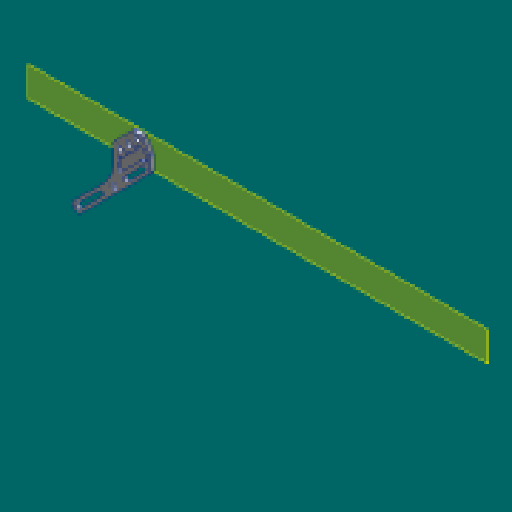
# Autodesk Inventor part: IntakeRampSidePlate
Saved by Autodesk Inventor 2023.1 (Build 271208000, 208)
## iProperties
Created: 2022-11-11
Part Number: IntakeRampSidePlate
Material: Aluminum 6061
Document SubType Name: Modeling
Designer: zac-h
Density: 2.7 g/cm^3
Appearance: Aluminum - Flat
Author: zac-h
Autodesk Inventor part; units mm, degrees
(part 1 of 2)
ref_plane "YZ Plane" through (0, 0, 0) normal (1, 0, 0) x (0, 1, 0)
ref_plane "XZ Plane" through (0, 0, 0) normal (0, 1, 0) x (-1, 0, 0)
ref_plane "XY Plane" through (0, 0, 0) normal (0, 0, 1) x (1, 0, 0)
ref_plane "Work Plane1" through (0, 0, 0) normal (0, 0, 1) x (1, 0, 0)
sketch "Sketch1" plane through (0, 0, 0) normal (0, 0, 1) x (1, 0, 0)
  line L0 (-428.9886, 23.7237) -> (-428.9886, 20.1169) projected
  arc A0 (-429.4966, 19.6089) -> (-428.9886, 20.1169) centre (-429.4966, 20.1169) ccw projected
  line L1 (-429.4966, 19.6089) -> (-433.1034, 19.6089) projected
  arc A1 (-433.6114, 20.1169) -> (-433.1034, 19.6089) centre (-433.1034, 20.1169) ccw projected
  line L2 (-433.6114, 20.1169) -> (-433.6114, 23.7237) projected
  arc A2 (-433.1034, 24.2317) -> (-433.6114, 23.7237) centre (-433.1034, 23.7237) ccw projected
  line L3 (-433.1034, 24.2317) -> (-429.4966, 24.2317) projected
  arc A3 (-428.9886, 23.7237) -> (-429.4966, 24.2317) centre (-429.4966, 23.7237) ccw projected
  line L4 (-416.2886, 23.7237) -> (-416.2886, 20.1169) projected
  arc A4 (-416.7966, 19.6089) -> (-416.2886, 20.1169) centre (-416.7966, 20.1169) ccw projected
  line L5 (-416.7966, 19.6089) -> (-420.4034, 19.6089) projected
  arc A5 (-420.9114, 20.1169) -> (-420.4034, 19.6089) centre (-420.4034, 20.1169) ccw projected
  line L6 (-420.9114, 20.1169) -> (-420.9114, 23.7237) projected
  arc A6 (-420.4034, 24.2317) -> (-420.9114, 23.7237) centre (-420.4034, 23.7237) ccw projected
  line L7 (-420.4034, 24.2317) -> (-416.7966, 24.2317) projected
  arc A7 (-416.2886, 23.7237) -> (-416.7966, 24.2317) centre (-416.7966, 23.7237) ccw projected
  line L8 (-403.5886, 23.7237) -> (-403.5886, 20.1169) projected
  arc A8 (-404.0966, 19.6089) -> (-403.5886, 20.1169) centre (-404.0966, 20.1169) ccw projected
  line L9 (-404.0966, 19.6089) -> (-407.7034, 19.6089) projected
  arc A9 (-408.2114, 20.1169) -> (-407.7034, 19.6089) centre (-407.7034, 20.1169) ccw projected
  line L10 (-408.2114, 20.1169) -> (-408.2114, 23.7237) projected
  arc A10 (-407.7034, 24.2317) -> (-408.2114, 23.7237) centre (-407.7034, 23.7237) ccw projected
  line L11 (-407.7034, 24.2317) -> (-404.0966, 24.2317) projected
  arc A11 (-403.5886, 23.7237) -> (-404.0966, 24.2317) centre (-404.0966, 23.7237) ccw projected
  line L12 (-390.8886, 23.7237) -> (-390.8886, 20.1169) projected
  arc A12 (-391.3966, 19.6089) -> (-390.8886, 20.1169) centre (-391.3966, 20.1169) ccw projected
  line L13 (-391.3966, 19.6089) -> (-395.0034, 19.6089) projected
  arc A13 (-395.5114, 20.1169) -> (-395.0034, 19.6089) centre (-395.0034, 20.1169) ccw projected
  line L14 (-395.5114, 20.1169) -> (-395.5114, 23.7237) projected
  arc A14 (-395.0034, 24.2317) -> (-395.5114, 23.7237) centre (-395.0034, 23.7237) ccw projected
  line L15 (-395.0034, 24.2317) -> (-391.3966, 24.2317) projected
  arc A15 (-390.8886, 23.7237) -> (-391.3966, 24.2317) centre (-391.3966, 23.7237) ccw projected
  line L16 (-378.1886, 23.7237) -> (-378.1886, 20.1169) projected
  arc A16 (-378.6966, 19.6089) -> (-378.1886, 20.1169) centre (-378.6966, 20.1169) ccw projected
  line L17 (-378.6966, 19.6089) -> (-382.3034, 19.6089) projected
  arc A17 (-382.8114, 20.1169) -> (-382.3034, 19.6089) centre (-382.3034, 20.1169) ccw projected
  line L18 (-382.8114, 20.1169) -> (-382.8114, 23.7237) projected
  arc A18 (-382.3034, 24.2317) -> (-382.8114, 23.7237) centre (-382.3034, 23.7237) ccw projected
  line L19 (-382.3034, 24.2317) -> (-378.6966, 24.2317) projected
  arc A19 (-378.1886, 23.7237) -> (-378.6966, 24.2317) centre (-378.6966, 23.7237) ccw projected
  line L20 (-365.4886, 23.7237) -> (-365.4886, 20.1169) projected
  arc A20 (-365.9966, 19.6089) -> (-365.4886, 20.1169) centre (-365.9966, 20.1169) ccw projected
  line L21 (-365.9966, 19.6089) -> (-369.6034, 19.6089) projected
  arc A21 (-370.1114, 20.1169) -> (-369.6034, 19.6089) centre (-369.6034, 20.1169) ccw projected
  line L22 (-370.1114, 20.1169) -> (-370.1114, 23.7237) projected
  arc A22 (-369.6034, 24.2317) -> (-370.1114, 23.7237) centre (-369.6034, 23.7237) ccw projected
  line L23 (-369.6034, 24.2317) -> (-365.9966, 24.2317) projected
  arc A23 (-365.4886, 23.7237) -> (-365.9966, 24.2317) centre (-365.9966, 23.7237) ccw projected
  line L24 (-352.7886, 23.7237) -> (-352.7886, 20.1169) projected
  arc A24 (-353.2966, 19.6089) -> (-352.7886, 20.1169) centre (-353.2966, 20.1169) ccw projected
  line L25 (-353.2966, 19.6089) -> (-356.9034, 19.6089) projected
  arc A25 (-357.4114, 20.1169) -> (-356.9034, 19.6089) centre (-356.9034, 20.1169) ccw projected
  line L26 (-357.4114, 20.1169) -> (-357.4114, 23.7237) projected
  arc A26 (-356.9034, 24.2317) -> (-357.4114, 23.7237) centre (-356.9034, 23.7237) ccw projected
  line L27 (-356.9034, 24.2317) -> (-353.2966, 24.2317) projected
  arc A27 (-352.7886, 23.7237) -> (-353.2966, 24.2317) centre (-353.2966, 23.7237) ccw projected
  line L28 (-340.0886, 23.7237) -> (-340.0886, 20.1169) projected
  arc A28 (-340.5966, 19.6089) -> (-340.0886, 20.1169) centre (-340.5966, 20.1169) ccw projected
  line L29 (-340.5966, 19.6089) -> (-344.2034, 19.6089) projected
  arc A29 (-344.7114, 20.1169) -> (-344.2034, 19.6089) centre (-344.2034, 20.1169) ccw projected
  line L30 (-344.7114, 20.1169) -> (-344.7114, 23.7237) projected
  arc A30 (-344.2034, 24.2317) -> (-344.7114, 23.7237) centre (-344.2034, 23.7237) ccw projected
  line L31 (-344.2034, 24.2317) -> (-340.5966, 24.2317) projected
  arc A31 (-340.0886, 23.7237) -> (-340.5966, 24.2317) centre (-340.5966, 23.7237) ccw projected
  line L32 (-327.3886, 23.7237) -> (-327.3886, 20.1169) projected
  arc A32 (-327.8966, 19.6089) -> (-327.3886, 20.1169) centre (-327.8966, 20.1169) ccw projected
  line L33 (-327.8966, 19.6089) -> (-331.5034, 19.6089) projected
  arc A33 (-332.0114, 20.1169) -> (-331.5034, 19.6089) centre (-331.5034, 20.1169) ccw projected
  line L34 (-332.0114, 20.1169) -> (-332.0114, 23.7237) projected
  arc A34 (-331.5034, 24.2317) -> (-332.0114, 23.7237) centre (-331.5034, 23.7237) ccw projected
  line L35 (-331.5034, 24.2317) -> (-327.8966, 24.2317) projected
  arc A35 (-327.3886, 23.7237) -> (-327.8966, 24.2317) centre (-327.8966, 23.7237) ccw projected
  line L36 (-314.6886, 23.7237) -> (-314.6886, 20.1169) projected
  arc A36 (-315.1966, 19.6089) -> (-314.6886, 20.1169) centre (-315.1966, 20.1169) ccw projected
  line L37 (-315.1966, 19.6089) -> (-318.8034, 19.6089) projected
  arc A37 (-319.3114, 20.1169) -> (-318.8034, 19.6089) centre (-318.8034, 20.1169) ccw projected
  line L38 (-319.3114, 20.1169) -> (-319.3114, 23.7237) projected
  arc A38 (-318.8034, 24.2317) -> (-319.3114, 23.7237) centre (-318.8034, 23.7237) ccw projected
  line L39 (-318.8034, 24.2317) -> (-315.1966, 24.2317) projected
  arc A39 (-314.6886, 23.7237) -> (-315.1966, 24.2317) centre (-315.1966, 23.7237) ccw projected
  line L40 (-301.9886, 23.7237) -> (-301.9886, 20.1169) projected
  arc A40 (-302.4966, 19.6089) -> (-301.9886, 20.1169) centre (-302.4966, 20.1169) ccw projected
  line L41 (-302.4966, 19.6089) -> (-306.1034, 19.6089) projected
  arc A41 (-306.6114, 20.1169) -> (-306.1034, 19.6089) centre (-306.1034, 20.1169) ccw projected
  line L42 (-306.6114, 20.1169) -> (-306.6114, 23.7237) projected
  arc A42 (-306.1034, 24.2317) -> (-306.6114, 23.7237) centre (-306.1034, 23.7237) ccw projected
  line L43 (-306.1034, 24.2317) -> (-302.4966, 24.2317) projected
  arc A43 (-301.9886, 23.7237) -> (-302.4966, 24.2317) centre (-302.4966, 23.7237) ccw projected
  line L44 (-289.2886, 23.7237) -> (-289.2886, 20.1169) projected
  arc A44 (-289.7966, 19.6089) -> (-289.2886, 20.1169) centre (-289.7966, 20.1169) ccw projected
  line L45 (-289.7966, 19.6089) -> (-293.4034, 19.6089) projected
  arc A45 (-293.9114, 20.1169) -> (-293.4034, 19.6089) centre (-293.4034, 20.1169) ccw projected
  line L46 (-293.9114, 20.1169) -> (-293.9114, 23.7237) projected
  arc A46 (-293.4034, 24.2317) -> (-293.9114, 23.7237) centre (-293.4034, 23.7237) ccw projected
  line L47 (-293.4034, 24.2317) -> (-289.7966, 24.2317) projected
  arc A47 (-289.2886, 23.7237) -> (-289.7966, 24.2317) centre (-289.7966, 23.7237) ccw projected
  line L48 (-276.5886, 23.7237) -> (-276.5886, 20.1169) projected
  arc A48 (-277.0966, 19.6089) -> (-276.5886, 20.1169) centre (-277.0966, 20.1169) ccw projected
  line L49 (-277.0966, 19.6089) -> (-280.7034, 19.6089) projected
  arc A49 (-281.2114, 20.1169) -> (-280.7034, 19.6089) centre (-280.7034, 20.1169) ccw projected
  line L50 (-281.2114, 20.1169) -> (-281.2114, 23.7237) projected
  arc A50 (-280.7034, 24.2317) -> (-281.2114, 23.7237) centre (-280.7034, 23.7237) ccw projected
  line L51 (-280.7034, 24.2317) -> (-277.0966, 24.2317) projected
  arc A51 (-276.5886, 23.7237) -> (-277.0966, 24.2317) centre (-277.0966, 23.7237) ccw projected
  line L52 (-263.8886, 23.7237) -> (-263.8886, 20.1169) projected
  arc A52 (-264.3966, 19.6089) -> (-263.8886, 20.1169) centre (-264.3966, 20.1169) ccw projected
  line L53 (-264.3966, 19.6089) -> (-268.0034, 19.6089) projected
  arc A53 (-268.5114, 20.1169) -> (-268.0034, 19.6089) centre (-268.0034, 20.1169) ccw projected
  line L54 (-268.5114, 20.1169) -> (-268.5114, 23.7237) projected
  arc A54 (-268.0034, 24.2317) -> (-268.5114, 23.7237) centre (-268.0034, 23.7237) ccw projected
  line L55 (-268.0034, 24.2317) -> (-264.3966, 24.2317) projected
  arc A55 (-263.8886, 23.7237) -> (-264.3966, 24.2317) centre (-264.3966, 23.7237) ccw projected
  line L56 (-251.1886, 23.7237) -> (-251.1886, 20.1169) projected
  arc A56 (-251.6966, 19.6089) -> (-251.1886, 20.1169) centre (-251.6966, 20.1169) ccw projected
  line L57 (-251.6966, 19.6089) -> (-255.3034, 19.6089) projected
  arc A57 (-255.8114, 20.1169) -> (-255.3034, 19.6089) centre (-255.3034, 20.1169) ccw projected
  line L58 (-255.8114, 20.1169) -> (-255.8114, 23.7237) projected
  arc A58 (-255.3034, 24.2317) -> (-255.8114, 23.7237) centre (-255.3034, 23.7237) ccw projected
  line L59 (-255.3034, 24.2317) -> (-251.6966, 24.2317) projected
  arc A59 (-251.1886, 23.7237) -> (-251.6966, 24.2317) centre (-251.6966, 23.7237) ccw projected
  line L60 (-238.4886, 23.7237) -> (-238.4886, 20.1169) projected
  arc A60 (-238.9966, 19.6089) -> (-238.4886, 20.1169) centre (-238.9966, 20.1169) ccw projected
  line L61 (-238.9966, 19.6089) -> (-242.6034, 19.6089) projected
  arc A61 (-243.1114, 20.1169) -> (-242.6034, 19.6089) centre (-242.6034, 20.1169) ccw projected
  line L62 (-243.1114, 20.1169) -> (-243.1114, 23.7237) projected
  arc A62 (-242.6034, 24.2317) -> (-243.1114, 23.7237) centre (-242.6034, 23.7237) ccw projected
  line L63 (-242.6034, 24.2317) -> (-238.9966, 24.2317) projected
  arc A63 (-238.4886, 23.7237) -> (-238.9966, 24.2317) centre (-238.9966, 23.7237) ccw projected
  line L64 (-225.7886, 23.7237) -> (-225.7886, 20.1169) projected
  arc A64 (-226.2966, 19.6089) -> (-225.7886, 20.1169) centre (-226.2966, 20.1169) ccw projected
  line L65 (-226.2966, 19.6089) -> (-229.9034, 19.6089) projected
  arc A65 (-230.4114, 20.1169) -> (-229.9034, 19.6089) centre (-229.9034, 20.1169) ccw projected
  line L66 (-230.4114, 20.1169) -> (-230.4114, 23.7237) projected
  arc A66 (-229.9034, 24.2317) -> (-230.4114, 23.7237) centre (-229.9034, 23.7237) ccw projected
  line L67 (-229.9034, 24.2317) -> (-226.2966, 24.2317) projected
  arc A67 (-225.7886, 23.7237) -> (-226.2966, 24.2317) centre (-226.2966, 23.7237) ccw projected
  line L68 (-213.0886, 23.7237) -> (-213.0886, 20.1169) projected
  arc A68 (-213.5966, 19.6089) -> (-213.0886, 20.1169) centre (-213.5966, 20.1169) ccw projected
  line L69 (-213.5966, 19.6089) -> (-217.2034, 19.6089) projected
  arc A69 (-217.7114, 20.1169) -> (-217.2034, 19.6089) centre (-217.2034, 20.1169) ccw projected
  line L70 (-217.7114, 20.1169) -> (-217.7114, 23.7237) projected
  arc A70 (-217.2034, 24.2317) -> (-217.7114, 23.7237) centre (-217.2034, 23.7237) ccw projected
  line L71 (-217.2034, 24.2317) -> (-213.5966, 24.2317) projected
  arc A71 (-213.0886, 23.7237) -> (-213.5966, 24.2317) centre (-213.5966, 23.7237) ccw projected
  line L72 (-200.3886, 23.7237) -> (-200.3886, 20.1169) projected
  arc A72 (-200.8966, 19.6089) -> (-200.3886, 20.1169) centre (-200.8966, 20.1169) ccw projected
  line L73 (-200.8966, 19.6089) -> (-204.5034, 19.6089) projected
  arc A73 (-205.0114, 20.1169) -> (-204.5034, 19.6089) centre (-204.5034, 20.1169) ccw projected
  line L74 (-205.0114, 20.1169) -> (-205.0114, 23.7237) projected
  arc A74 (-204.5034, 24.2317) -> (-205.0114, 23.7237) centre (-204.5034, 23.7237) ccw projected
  line L75 (-204.5034, 24.2317) -> (-200.8966, 24.2317) projected
  arc A75 (-200.3886, 23.7237) -> (-200.8966, 24.2317) centre (-200.8966, 23.7237) ccw projected
  line L76 (-187.6886, 23.7237) -> (-187.6886, 20.1169) projected
  arc A76 (-188.1966, 19.6089) -> (-187.6886, 20.1169) centre (-188.1966, 20.1169) ccw projected
  line L77 (-188.1966, 19.6089) -> (-191.8034, 19.6089) projected
  arc A77 (-192.3114, 20.1169) -> (-191.8034, 19.6089) centre (-191.8034, 20.1169) ccw projected
  line L78 (-192.3114, 20.1169) -> (-192.3114, 23.7237) projected
  arc A78 (-191.8034, 24.2317) -> (-192.3114, 23.7237) centre (-191.8034, 23.7237) ccw projected
  line L79 (-191.8034, 24.2317) -> (-188.1966, 24.2317) projected
  arc A79 (-187.6886, 23.7237) -> (-188.1966, 24.2317) centre (-188.1966, 23.7237) ccw projected
  line L80 (-174.9886, 23.7237) -> (-174.9886, 20.1169) projected
  arc A80 (-175.4966, 19.6089) -> (-174.9886, 20.1169) centre (-175.4966, 20.1169) ccw projected
  line L81 (-175.4966, 19.6089) -> (-179.1034, 19.6089) projected
  arc A81 (-179.6114, 20.1169) -> (-179.1034, 19.6089) centre (-179.1034, 20.1169) ccw projected
  line L82 (-179.6114, 20.1169) -> (-179.6114, 23.7237) projected
  arc A82 (-179.1034, 24.2317) -> (-179.6114, 23.7237) centre (-179.1034, 23.7237) ccw projected
  line L83 (-179.1034, 24.2317) -> (-175.4966, 24.2317) projected
  arc A83 (-174.9886, 23.7237) -> (-175.4966, 24.2317) centre (-175.4966, 23.7237) ccw projected
  line L84 (-162.2886, 23.7237) -> (-162.2886, 20.1169) projected
  arc A84 (-162.7966, 19.6089) -> (-162.2886, 20.1169) centre (-162.7966, 20.1169) ccw projected
  line L85 (-162.7966, 19.6089) -> (-166.4034, 19.6089) projected
  arc A85 (-166.9114, 20.1169) -> (-166.4034, 19.6089) centre (-166.4034, 20.1169) ccw projected
  line L86 (-166.9114, 20.1169) -> (-166.9114, 23.7237) projected
  arc A86 (-166.4034, 24.2317) -> (-166.9114, 23.7237) centre (-166.4034, 23.7237) ccw projected
  line L87 (-166.4034, 24.2317) -> (-162.7966, 24.2317) projected
  arc A87 (-162.2886, 23.7237) -> (-162.7966, 24.2317) centre (-162.7966, 23.7237) ccw projected
  line L88 (-149.5886, 23.7237) -> (-149.5886, 20.1169) projected
  arc A88 (-150.0966, 19.6089) -> (-149.5886, 20.1169) centre (-150.0966, 20.1169) ccw projected
  line L89 (-150.0966, 19.6089) -> (-153.7034, 19.6089) projected
  arc A89 (-154.2114, 20.1169) -> (-153.7034, 19.6089) centre (-153.7034, 20.1169) ccw projected
  line L90 (-154.2114, 20.1169) -> (-154.2114, 23.7237) projected
  arc A90 (-153.7034, 24.2317) -> (-154.2114, 23.7237) centre (-153.7034, 23.7237) ccw projected
  line L91 (-153.7034, 24.2317) -> (-150.0966, 24.2317) projected
  arc A91 (-149.5886, 23.7237) -> (-150.0966, 24.2317) centre (-150.0966, 23.7237) ccw projected
  line L92 (-136.8886, 23.7237) -> (-136.8886, 20.1169) projected
  arc A92 (-137.3966, 19.6089) -> (-136.8886, 20.1169) centre (-137.3966, 20.1169) ccw projected
  line L93 (-137.3966, 19.6089) -> (-141.0034, 19.6089) projected
  arc A93 (-141.5114, 20.1169) -> (-141.0034, 19.6089) centre (-141.0034, 20.1169) ccw projected
  line L94 (-141.5114, 20.1169) -> (-141.5114, 23.7237) projected
  arc A94 (-141.0034, 24.2317) -> (-141.5114, 23.7237) centre (-141.0034, 23.7237) ccw projected
  line L95 (-141.0034, 24.2317) -> (-137.3966, 24.2317) projected
  arc A95 (-136.8886, 23.7237) -> (-137.3966, 24.2317) centre (-137.3966, 23.7237) ccw projected
  line L96 (-126.5, 19.6089) -> (-126.5, 12.6321) projected
  line L97 (-126.5, 19.6089) -> (-128.3034, 19.6089) projected
  arc A96 (-128.8114, 20.1169) -> (-128.3034, 19.6089) centre (-128.3034, 20.1169) ccw projected
  line L98 (-128.8114, 20.1169) -> (-128.8114, 23.7237) projected
  arc A97 (-128.3034, 24.2317) -> (-128.8114, 23.7237) centre (-128.3034, 23.7237) ccw projected
  line L99 (-128.3034, 24.2317) -> (-126.5, 24.2317) projected
  line L100 (-126.5, 31.2085) -> (-126.5, 24.2317) projected
  line L101 (-126.5, 31.2085) -> (-127.5242, 32.2327) projected
  line L102 (-127.5242, 32.2327) -> (-188.9758, 32.2327) projected
  line L103 (-190, 31.2085) -> (-188.9758, 32.2327) projected
  line L104 (-190, 31.2085) -> (-191.0242, 32.2327) projected
  line L105 (-191.0242, 32.2327) -> (-252.4758, 32.2327) projected
  line L106 (-253.5, 31.2085) -> (-252.4758, 32.2327) projected
  line L107 (-253.5, 31.2085) -> (-254.5242, 32.2327) projected
  line L108 (-254.5242, 32.2327) -> (-315.9758, 32.2327) projected
  line L109 (-317, 31.2085) -> (-315.9758, 32.2327) projected
  line L110 (-317, 31.2085) -> (-318.0242, 32.2327) projected
  line L111 (-318.0242, 32.2327) -> (-379.4758, 32.2327) projected
  line L112 (-379.4758, 32.2327) -> (-380.5, 31.2085) projected
  line L113 (-380.5, 31.2085) -> (-381.5242, 32.2327) projected
  line L114 (-381.5242, 32.2327) -> (-444, 32.2327) projected
  line L115 (-444, 32.2327) -> (-444, 11.6079) projected
  line L116 (-444, 11.6079) -> (-381.5242, 11.6079) projected
  line L117 (-381.5242, 11.6079) -> (-380.5, 12.6321) projected
  line L118 (-380.5, 12.6321) -> (-379.4758, 11.6079) projected
  line L119 (-379.4758, 11.6079) -> (-318.0242, 11.6079) projected
  line L120 (-317, 12.6321) -> (-318.0242, 11.6079) projected
  line L121 (-317, 12.6321) -> (-315.9758, 11.6079) projected
  line L122 (-315.9758, 11.6079) -> (-254.5242, 11.6079) projected
  line L123 (-253.5, 12.6321) -> (-254.5242, 11.6079) projected
  line L124 (-253.5, 12.6321) -> (-252.4758, 11.6079) projected
  line L125 (-252.4758, 11.6079) -> (-191.0242, 11.6079) projected
  line L126 (-190, 12.6321) -> (-191.0242, 11.6079) projected
  line L127 (-190, 12.6321) -> (-188.9758, 11.6079) projected
  line L128 (-188.9758, 11.6079) -> (-127.5242, 11.6079) projected
  line L129 (-126.5, 12.6321) -> (-127.5242, 11.6079) projected
  line L130 (-435.3386, 30.0737) -> (-435.3386, 26.4669) projected
  arc A98 (-435.8466, 25.9589) -> (-435.3386, 26.4669) centre (-435.8466, 26.4669) ccw projected
  line L131 (-435.8466, 25.9589) -> (-439.4534, 25.9589) projected
  arc A99 (-439.9614, 26.4669) -> (-439.4534, 25.9589) centre (-439.4534, 26.4669) ccw projected
  line L132 (-439.9614, 26.4669) -> (-439.9614, 30.0737) projected
  arc A100 (-439.4534, 30.5817) -> (-439.9614, 30.0737) centre (-439.4534, 30.0737) ccw projected
  line L133 (-439.4534, 30.5817) -> (-435.8466, 30.5817) projected
  arc A101 (-435.3386, 30.0737) -> (-435.8466, 30.5817) centre (-435.8466, 30.0737) ccw projected
  line L134 (-435.3386, 17.3737) -> (-435.3386, 13.7669) projected
  arc A102 (-435.8466, 13.2589) -> (-435.3386, 13.7669) centre (-435.8466, 13.7669) ccw projected
  line L135 (-435.8466, 13.2589) -> (-439.4534, 13.2589) projected
  arc A103 (-439.9614, 13.7669) -> (-439.4534, 13.2589) centre (-439.4534, 13.7669) ccw projected
  line L136 (-439.9614, 13.7669) -> (-439.9614, 17.3737) projected
  arc A104 (-439.4534, 17.8817) -> (-439.9614, 17.3737) centre (-439.4534, 17.3737) ccw projected
  line L137 (-439.4534, 17.8817) -> (-435.8466, 17.8817) projected
  arc A105 (-435.3386, 17.3737) -> (-435.8466, 17.8817) centre (-435.8466, 17.3737) ccw projected
  line L138 (-427.2614, 13.7669) -> (-427.2614, 17.3737) projected
  arc A106 (-426.7534, 17.8817) -> (-427.2614, 17.3737) centre (-426.7534, 17.3737) ccw projected
  line L139 (-426.7534, 17.8817) -> (-423.1466, 17.8817) projected
  arc A107 (-422.6386, 17.3737) -> (-423.1466, 17.8817) centre (-423.1466, 17.3737) ccw projected
  line L140 (-422.6386, 17.3737) -> (-422.6386, 13.7669) projected
  arc A108 (-423.1466, 13.2589) -> (-422.6386, 13.7669) centre (-423.1466, 13.7669) ccw projected
  line L141 (-423.1466, 13.2589) -> (-426.7534, 13.2589) projected
  arc A109 (-427.2614, 13.7669) -> (-426.7534, 13.2589) centre (-426.7534, 13.7669) ccw projected
  line L142 (-414.5614, 13.7669) -> (-414.5614, 17.3737) projected
  arc A110 (-414.0534, 17.8817) -> (-414.5614, 17.3737) centre (-414.0534, 17.3737) ccw projected
  line L143 (-414.0534, 17.8817) -> (-410.4466, 17.8817) projected
  arc A111 (-409.9386, 17.3737) -> (-410.4466, 17.8817) centre (-410.4466, 17.3737) ccw projected
  line L144 (-409.9386, 17.3737) -> (-409.9386, 13.7669) projected
  arc A112 (-410.4466, 13.2589) -> (-409.9386, 13.7669) centre (-410.4466, 13.7669) ccw projected
  line L145 (-410.4466, 13.2589) -> (-414.0534, 13.2589) projected
  arc A113 (-414.5614, 13.7669) -> (-414.0534, 13.2589) centre (-414.0534, 13.7669) ccw projected
  line L146 (-401.8614, 13.7669) -> (-401.8614, 17.3737) projected
  arc A114 (-401.3534, 17.8817) -> (-401.8614, 17.3737) centre (-401.3534, 17.3737) ccw projected
  line L147 (-401.3534, 17.8817) -> (-397.7466, 17.8817) projected
  arc A115 (-397.2386, 17.3737) -> (-397.7466, 17.8817) centre (-397.7466, 17.3737) ccw projected
  line L148 (-397.2386, 17.3737) -> (-397.2386, 13.7669) projected
  arc A116 (-397.7466, 13.2589) -> (-397.2386, 13.7669) centre (-397.7466, 13.7669) ccw projected
  line L149 (-397.7466, 13.2589) -> (-401.3534, 13.2589) projected
  arc A117 (-401.8614, 13.7669) -> (-401.3534, 13.2589) centre (-401.3534, 13.7669) ccw projected
  line L150 (-389.1614, 13.7669) -> (-389.1614, 17.3737) projected
  arc A118 (-388.6534, 17.8817) -> (-389.1614, 17.3737) centre (-388.6534, 17.3737) ccw projected
  line L151 (-388.6534, 17.8817) -> (-385.0466, 17.8817) projected
  arc A119 (-384.5386, 17.3737) -> (-385.0466, 17.8817) centre (-385.0466, 17.3737) ccw projected
  line L152 (-384.5386, 17.3737) -> (-384.5386, 13.7669) projected
  arc A120 (-385.0466, 13.2589) -> (-384.5386, 13.7669) centre (-385.0466, 13.7669) ccw projected
  line L153 (-385.0466, 13.2589) -> (-388.6534, 13.2589) projected
  arc A121 (-389.1614, 13.7669) -> (-388.6534, 13.2589) centre (-388.6534, 13.7669) ccw projected
  line L154 (-376.4614, 13.7669) -> (-376.4614, 17.3737) projected
  arc A122 (-375.9534, 17.8817) -> (-376.4614, 17.3737) centre (-375.9534, 17.3737) ccw projected
  line L155 (-375.9534, 17.8817) -> (-372.3466, 17.8817) projected
  arc A123 (-371.8386, 17.3737) -> (-372.3466, 17.8817) centre (-372.3466, 17.3737) ccw projected
  line L156 (-371.8386, 17.3737) -> (-371.8386, 13.7669) projected
  arc A124 (-372.3466, 13.2589) -> (-371.8386, 13.7669) centre (-372.3466, 13.7669) ccw projected
  line L157 (-372.3466, 13.2589) -> (-375.9534, 13.2589) projected
  arc A125 (-376.4614, 13.7669) -> (-375.9534, 13.2589) centre (-375.9534, 13.7669) ccw projected
  line L158 (-363.7614, 13.7669) -> (-363.7614, 17.3737) projected
  arc A126 (-363.2534, 17.8817) -> (-363.7614, 17.3737) centre (-363.2534, 17.3737) ccw projected
  line L159 (-363.2534, 17.8817) -> (-359.6466, 17.8817) projected
  arc A127 (-359.1386, 17.3737) -> (-359.6466, 17.8817) centre (-359.6466, 17.3737) ccw projected
  line L160 (-359.1386, 17.3737) -> (-359.1386, 13.7669) projected
  arc A128 (-359.6466, 13.2589) -> (-359.1386, 13.7669) centre (-359.6466, 13.7669) ccw projected
  line L161 (-359.6466, 13.2589) -> (-363.2534, 13.2589) projected
  arc A129 (-363.7614, 13.7669) -> (-363.2534, 13.2589) centre (-363.2534, 13.7669) ccw projected
  line L162 (-351.0614, 13.7669) -> (-351.0614, 17.3737) projected
  arc A130 (-350.5534, 17.8817) -> (-351.0614, 17.3737) centre (-350.5534, 17.3737) ccw projected
  line L163 (-350.5534, 17.8817) -> (-346.9466, 17.8817) projected
  arc A131 (-346.4386, 17.3737) -> (-346.9466, 17.8817) centre (-346.9466, 17.3737) ccw projected
  line L164 (-346.4386, 17.3737) -> (-346.4386, 13.7669) projected
  arc A132 (-346.9466, 13.2589) -> (-346.4386, 13.7669) centre (-346.9466, 13.7669) ccw projected
  line L165 (-346.9466, 13.2589) -> (-350.5534, 13.2589) projected
  arc A133 (-351.0614, 13.7669) -> (-350.5534, 13.2589) centre (-350.5534, 13.7669) ccw projected
  line L166 (-338.3614, 13.7669) -> (-338.3614, 17.3737) projected
  arc A134 (-337.8534, 17.8817) -> (-338.3614, 17.3737) centre (-337.8534, 17.3737) ccw projected
  line L167 (-337.8534, 17.8817) -> (-334.2466, 17.8817) projected
  arc A135 (-333.7386, 17.3737) -> (-334.2466, 17.8817) centre (-334.2466, 17.3737) ccw projected
  line L168 (-333.7386, 17.3737) -> (-333.7386, 13.7669) projected
  arc A136 (-334.2466, 13.2589) -> (-333.7386, 13.7669) centre (-334.2466, 13.7669) ccw projected
  line L169 (-334.2466, 13.2589) -> (-337.8534, 13.2589) projected
  arc A137 (-338.3614, 13.7669) -> (-337.8534, 13.2589) centre (-337.8534, 13.7669) ccw projected
  line L170 (-325.6614, 13.7669) -> (-325.6614, 17.3737) projected
  arc A138 (-325.1534, 17.8817) -> (-325.6614, 17.3737) centre (-325.1534, 17.3737) ccw projected
  line L171 (-325.1534, 17.8817) -> (-321.5466, 17.8817) projected
  arc A139 (-321.0386, 17.3737) -> (-321.5466, 17.8817) centre (-321.5466, 17.3737) ccw projected
  line L172 (-321.0386, 17.3737) -> (-321.0386, 13.7669) projected
  arc A140 (-321.5466, 13.2589) -> (-321.0386, 13.7669) centre (-321.5466, 13.7669) ccw projected
  line L173 (-321.5466, 13.2589) -> (-325.1534, 13.2589) projected
  arc A141 (-325.6614, 13.7669) -> (-325.1534, 13.2589) centre (-325.1534, 13.7669) ccw projected
  line L174 (-312.9614, 13.7669) -> (-312.9614, 17.3737) projected
  arc A142 (-312.4534, 17.8817) -> (-312.9614, 17.3737) centre (-312.4534, 17.3737) ccw projected
  line L175 (-312.4534, 17.8817) -> (-308.8466, 17.8817) projected
  arc A143 (-308.3386, 17.3737) -> (-308.8466, 17.8817) centre (-308.8466, 17.3737) ccw projected
  line L176 (-308.3386, 17.3737) -> (-308.3386, 13.7669) projected
  arc A144 (-308.8466, 13.2589) -> (-308.3386, 13.7669) centre (-308.8466, 13.7669) ccw projected
  line L177 (-308.8466, 13.2589) -> (-312.4534, 13.2589) projected
  arc A145 (-312.9614, 13.7669) -> (-312.4534, 13.2589) centre (-312.4534, 13.7669) ccw projected
  line L178 (-300.2614, 13.7669) -> (-300.2614, 17.3737) projected
  arc A146 (-299.7534, 17.8817) -> (-300.2614, 17.3737) centre (-299.7534, 17.3737) ccw projected
  line L179 (-299.7534, 17.8817) -> (-296.1466, 17.8817) projected
  arc A147 (-295.6386, 17.3737) -> (-296.1466, 17.8817) centre (-296.1466, 17.3737) ccw projected
  line L180 (-295.6386, 17.3737) -> (-295.6386, 13.7669) projected
  arc A148 (-296.1466, 13.2589) -> (-295.6386, 13.7669) centre (-296.1466, 13.7669) ccw projected
  line L181 (-296.1466, 13.2589) -> (-299.7534, 13.2589) projected
  arc A149 (-300.2614, 13.7669) -> (-299.7534, 13.2589) centre (-299.7534, 13.7669) ccw projected
  line L182 (-287.5614, 13.7669) -> (-287.5614, 17.3737) projected
  arc A150 (-287.0534, 17.8817) -> (-287.5614, 17.3737) centre (-287.0534, 17.3737) ccw projected
  line L183 (-287.0534, 17.8817) -> (-283.4466, 17.8817) projected
  arc A151 (-282.9386, 17.3737) -> (-283.4466, 17.8817) centre (-283.4466, 17.3737) ccw projected
  line L184 (-282.9386, 17.3737) -> (-282.9386, 13.7669) projected
  arc A152 (-283.4466, 13.2589) -> (-282.9386, 13.7669) centre (-283.4466, 13.7669) ccw projected
  line L185 (-283.4466, 13.2589) -> (-287.0534, 13.2589) projected
  arc A153 (-287.5614, 13.7669) -> (-287.0534, 13.2589) centre (-287.0534, 13.7669) ccw projected
  line L186 (-274.8614, 13.7669) -> (-274.8614, 17.3737) projected
  arc A154 (-274.3534, 17.8817) -> (-274.8614, 17.3737) centre (-274.3534, 17.3737) ccw projected
  line L187 (-274.3534, 17.8817) -> (-270.7466, 17.8817) projected
  arc A155 (-270.2386, 17.3737) -> (-270.7466, 17.8817) centre (-270.7466, 17.3737) ccw projected
  line L188 (-270.2386, 17.3737) -> (-270.2386, 13.7669) projected
  arc A156 (-270.7466, 13.2589) -> (-270.2386, 13.7669) centre (-270.7466, 13.7669) ccw projected
  line L189 (-270.7466, 13.2589) -> (-274.3534, 13.2589) projected
  arc A157 (-274.8614, 13.7669) -> (-274.3534, 13.2589) centre (-274.3534, 13.7669) ccw projected
  line L190 (-262.1614, 13.7669) -> (-262.1614, 17.3737) projected
  arc A158 (-261.6534, 17.8817) -> (-262.1614, 17.3737) centre (-261.6534, 17.3737) ccw projected
  line L191 (-261.6534, 17.8817) -> (-258.0466, 17.8817) projected
  arc A159 (-257.5386, 17.3737) -> (-258.0466, 17.8817) centre (-258.0466, 17.3737) ccw projected
  line L192 (-257.5386, 17.3737) -> (-257.5386, 13.7669) projected
  arc A160 (-258.0466, 13.2589) -> (-257.5386, 13.7669) centre (-258.0466, 13.7669) ccw projected
  line L193 (-258.0466, 13.2589) -> (-261.6534, 13.2589) projected
  arc A161 (-262.1614, 13.7669) -> (-261.6534, 13.2589) centre (-261.6534, 13.7669) ccw projected
  line L194 (-249.4614, 13.7669) -> (-249.4614, 17.3737) projected
  arc A162 (-248.9534, 17.8817) -> (-249.4614, 17.3737) centre (-248.9534, 17.3737) ccw projected
  line L195 (-248.9534, 17.8817) -> (-245.3466, 17.8817) projected
  arc A163 (-244.8386, 17.3737) -> (-245.3466, 17.8817) centre (-245.3466, 17.3737) ccw projected
  line L196 (-244.8386, 17.3737) -> (-244.8386, 13.7669) projected
  arc A164 (-245.3466, 13.2589) -> (-244.8386, 13.7669) centre (-245.3466, 13.7669) ccw projected
  line L197 (-245.3466, 13.2589) -> (-248.9534, 13.2589) projected
  arc A165 (-249.4614, 13.7669) -> (-248.9534, 13.2589) centre (-248.9534, 13.7669) ccw projected
  line L198 (-236.7614, 13.7669) -> (-236.7614, 17.3737) projected
  arc A166 (-236.2534, 17.8817) -> (-236.7614, 17.3737) centre (-236.2534, 17.3737) ccw projected
  line L199 (-236.2534, 17.8817) -> (-232.6466, 17.8817) projected
  arc A167 (-232.1386, 17.3737) -> (-232.6466, 17.8817) centre (-232.6466, 17.3737) ccw projected
  line L200 (-232.1386, 17.3737) -> (-232.1386, 13.7669) projected
  arc A168 (-232.6466, 13.2589) -> (-232.1386, 13.7669) centre (-232.6466, 13.7669) ccw projected
  line L201 (-232.6466, 13.2589) -> (-236.2534, 13.2589) projected
  arc A169 (-236.7614, 13.7669) -> (-236.2534, 13.2589) centre (-236.2534, 13.7669) ccw projected
  line L202 (-224.0614, 13.7669) -> (-224.0614, 17.3737) projected
  arc A170 (-223.5534, 17.8817) -> (-224.0614, 17.3737) centre (-223.5534, 17.3737) ccw projected
  line L203 (-223.5534, 17.8817) -> (-219.9466, 17.8817) projected
  arc A171 (-219.4386, 17.3737) -> (-219.9466, 17.8817) centre (-219.9466, 17.3737) ccw projected
  line L204 (-219.4386, 17.3737) -> (-219.4386, 13.7669) projected
  arc A172 (-219.9466, 13.2589) -> (-219.4386, 13.7669) centre (-219.9466, 13.7669) ccw projected
  line L205 (-219.9466, 13.2589) -> (-223.5534, 13.2589) projected
  arc A173 (-224.0614, 13.7669) -> (-223.5534, 13.2589) centre (-223.5534, 13.7669) ccw projected
  line L206 (-211.3614, 13.7669) -> (-211.3614, 17.3737) projected
  arc A174 (-210.8534, 17.8817) -> (-211.3614, 17.3737) centre (-210.8534, 17.3737) ccw projected
  line L207 (-210.8534, 17.8817) -> (-207.2466, 17.8817) projected
  arc A175 (-206.7386, 17.3737) -> (-207.2466, 17.8817) centre (-207.2466, 17.3737) ccw projected
  line L208 (-206.7386, 17.3737) -> (-206.7386, 13.7669) projected
  arc A176 (-207.2466, 13.2589) -> (-206.7386, 13.7669) centre (-207.2466, 13.7669) ccw projected
  line L209 (-207.2466, 13.2589) -> (-210.8534, 13.2589) projected
  arc A177 (-211.3614, 13.7669) -> (-210.8534, 13.2589) centre (-210.8534, 13.7669) ccw projected
  line L210 (-198.6614, 13.7669) -> (-198.6614, 17.3737) projected
  arc A178 (-198.1534, 17.8817) -> (-198.6614, 17.3737) centre (-198.1534, 17.3737) ccw projected
  line L211 (-198.1534, 17.8817) -> (-194.5466, 17.8817) projected
  arc A179 (-194.0386, 17.3737) -> (-194.5466, 17.8817) centre (-194.5466, 17.3737) ccw projected
  line L212 (-194.0386, 17.3737) -> (-194.0386, 13.7669) projected
  arc A180 (-194.5466, 13.2589) -> (-194.0386, 13.7669) centre (-194.5466, 13.7669) ccw projected
  line L213 (-194.5466, 13.2589) -> (-198.1534, 13.2589) projected
  arc A181 (-198.6614, 13.7669) -> (-198.1534, 13.2589) centre (-198.1534, 13.7669) ccw projected
  line L214 (-185.9614, 13.7669) -> (-185.9614, 17.3737) projected
  arc A182 (-185.4534, 17.8817) -> (-185.9614, 17.3737) centre (-185.4534, 17.3737) ccw projected
  line L215 (-185.4534, 17.8817) -> (-181.8466, 17.8817) projected
  arc A183 (-181.3386, 17.3737) -> (-181.8466, 17.8817) centre (-181.8466, 17.3737) ccw projected
  line L216 (-181.3386, 17.3737) -> (-181.3386, 13.7669) projected
  arc A184 (-181.8466, 13.2589) -> (-181.3386, 13.7669) centre (-181.8466, 13.7669) ccw projected
  line L217 (-181.8466, 13.2589) -> (-185.4534, 13.2589) projected
  arc A185 (-185.9614, 13.7669) -> (-185.4534, 13.2589) centre (-185.4534, 13.7669) ccw projected
  line L218 (-173.2614, 13.7669) -> (-173.2614, 17.3737) projected
  arc A186 (-172.7534, 17.8817) -> (-173.2614, 17.3737) centre (-172.7534, 17.3737) ccw projected
  line L219 (-172.7534, 17.8817) -> (-169.1466, 17.8817) projected
  arc A187 (-168.6386, 17.3737) -> (-169.1466, 17.8817) centre (-169.1466, 17.3737) ccw projected
  line L220 (-168.6386, 17.3737) -> (-168.6386, 13.7669) projected
  arc A188 (-169.1466, 13.2589) -> (-168.6386, 13.7669) centre (-169.1466, 13.7669) ccw projected
  line L221 (-169.1466, 13.2589) -> (-172.7534, 13.2589) projected
  arc A189 (-173.2614, 13.7669) -> (-172.7534, 13.2589) centre (-172.7534, 13.7669) ccw projected
  line L222 (-160.5614, 13.7669) -> (-160.5614, 17.3737) projected
  arc A190 (-160.0534, 17.8817) -> (-160.5614, 17.3737) centre (-160.0534, 17.3737) ccw projected
  line L223 (-160.0534, 17.8817) -> (-156.4466, 17.8817) projected
  arc A191 (-155.9386, 17.3737) -> (-156.4466, 17.8817) centre (-156.4466, 17.3737) ccw projected
  line L224 (-155.9386, 17.3737) -> (-155.9386, 13.7669) projected
  arc A192 (-156.4466, 13.2589) -> (-155.9386, 13.7669) centre (-156.4466, 13.7669) ccw projected
  line L225 (-156.4466, 13.2589) -> (-160.0534, 13.2589) projected
  arc A193 (-160.5614, 13.7669) -> (-160.0534, 13.2589) centre (-160.0534, 13.7669) ccw projected
  line L226 (-147.8614, 13.7669) -> (-147.8614, 17.3737) projected
  arc A194 (-147.3534, 17.8817) -> (-147.8614, 17.3737) centre (-147.3534, 17.3737) ccw projected
  line L227 (-147.3534, 17.8817) -> (-143.7466, 17.8817) projected
  arc A195 (-143.2386, 17.3737) -> (-143.7466, 17.8817) centre (-143.7466, 17.3737) ccw projected
  line L228 (-143.2386, 17.3737) -> (-143.2386, 13.7669) projected
  arc A196 (-143.7466, 13.2589) -> (-143.2386, 13.7669) centre (-143.7466, 13.7669) ccw projected
  line L229 (-143.7466, 13.2589) -> (-147.3534, 13.2589) projected
  arc A197 (-147.8614, 13.7669) -> (-147.3534, 13.2589) centre (-147.3534, 13.7669) ccw projected
  line L230 (-135.1614, 13.7669) -> (-135.1614, 17.3737) projected
  arc A198 (-134.6534, 17.8817) -> (-135.1614, 17.3737) centre (-134.6534, 17.3737) ccw projected
  line L231 (-134.6534, 17.8817) -> (-131.0466, 17.8817) projected
  arc A199 (-130.5386, 17.3737) -> (-131.0466, 17.8817) centre (-131.0466, 17.3737) ccw projected
  line L232 (-130.5386, 17.3737) -> (-130.5386, 13.7669) projected
  arc A200 (-131.0466, 13.2589) -> (-130.5386, 13.7669) centre (-131.0466, 13.7669) ccw projected
  line L233 (-131.0466, 13.2589) -> (-134.6534, 13.2589) projected
  arc A201 (-135.1614, 13.7669) -> (-134.6534, 13.2589) centre (-134.6534, 13.7669) ccw projected
  line L234 (-427.2614, 26.4669) -> (-427.2614, 30.0737) projected
  arc A202 (-426.7534, 30.5817) -> (-427.2614, 30.0737) centre (-426.7534, 30.0737) ccw projected
  line L235 (-426.7534, 30.5817) -> (-423.1466, 30.5817) projected
  arc A203 (-422.6386, 30.0737) -> (-423.1466, 30.5817) centre (-423.1466, 30.0737) ccw projected
  line L236 (-422.6386, 30.0737) -> (-422.6386, 26.4669) projected
  arc A204 (-423.1466, 25.9589) -> (-422.6386, 26.4669) centre (-423.1466, 26.4669) ccw projected
  line L237 (-423.1466, 25.9589) -> (-426.7534, 25.9589) projected
  arc A205 (-427.2614, 26.4669) -> (-426.7534, 25.9589) centre (-426.7534, 26.4669) ccw projected
  line L238 (-414.5614, 26.4669) -> (-414.5614, 30.0737) projected
  arc A206 (-414.0534, 30.5817) -> (-414.5614, 30.0737) centre (-414.0534, 30.0737) ccw projected
  line L239 (-414.0534, 30.5817) -> (-410.4466, 30.5817) projected
  arc A207 (-409.9386, 30.0737) -> (-410.4466, 30.5817) centre (-410.4466, 30.0737) ccw projected
  line L240 (-409.9386, 30.0737) -> (-409.9386, 26.4669) projected
  arc A208 (-410.4466, 25.9589) -> (-409.9386, 26.4669) centre (-410.4466, 26.4669) ccw projected
  line L241 (-410.4466, 25.9589) -> (-414.0534, 25.9589) projected
  arc A209 (-414.5614, 26.4669) -> (-414.0534, 25.9589) centre (-414.0534, 26.4669) ccw projected
  line L242 (-401.8614, 26.4669) -> (-401.8614, 30.0737) projected
  arc A210 (-401.3534, 30.5817) -> (-401.8614, 30.0737) centre (-401.3534, 30.0737) ccw projected
  line L243 (-401.3534, 30.5817) -> (-397.7466, 30.5817) projected
  arc A211 (-397.2386, 30.0737) -> (-397.7466, 30.5817) centre (-397.7466, 30.0737) ccw projected
  line L244 (-397.2386, 30.0737) -> (-397.2386, 26.4669) projected
  arc A212 (-397.7466, 25.9589) -> (-397.2386, 26.4669) centre (-397.7466, 26.4669) ccw projected
  line L245 (-397.7466, 25.9589) -> (-401.3534, 25.9589) projected
  arc A213 (-401.8614, 26.4669) -> (-401.3534, 25.9589) centre (-401.3534, 26.4669) ccw projected
  line L246 (-389.1614, 26.4669) -> (-389.1614, 30.0737) projected
  arc A214 (-388.6534, 30.5817) -> (-389.1614, 30.0737) centre (-388.6534, 30.0737) ccw projected
  line L247 (-388.6534, 30.5817) -> (-385.0466, 30.5817) projected
  arc A215 (-384.5386, 30.0737) -> (-385.0466, 30.5817) centre (-385.0466, 30.0737) ccw projected
  line L248 (-384.5386, 30.0737) -> (-384.5386, 26.4669) projected
  arc A216 (-385.0466, 25.9589) -> (-384.5386, 26.4669) centre (-385.0466, 26.4669) ccw projected
  line L249 (-385.0466, 25.9589) -> (-388.6534, 25.9589) projected
  arc A217 (-389.1614, 26.4669) -> (-388.6534, 25.9589) centre (-388.6534, 26.4669) ccw projected
  line L250 (-376.4614, 26.4669) -> (-376.4614, 30.0737) projected
  arc A218 (-375.9534, 30.5817) -> (-376.4614, 30.0737) centre (-375.9534, 30.0737) ccw projected
  line L251 (-375.9534, 30.5817) -> (-372.3466, 30.5817) projected
  arc A219 (-371.8386, 30.0737) -> (-372.3466, 30.5817) centre (-372.3466, 30.0737) ccw projected
  line L252 (-371.8386, 30.0737) -> (-371.8386, 26.4669) projected
  arc A220 (-372.3466, 25.9589) -> (-371.8386, 26.4669) centre (-372.3466, 26.4669) ccw projected
  line L253 (-372.3466, 25.9589) -> (-375.9534, 25.9589) projected
  arc A221 (-376.4614, 26.4669) -> (-375.9534, 25.9589) centre (-375.9534, 26.4669) ccw projected
  line L254 (-363.7614, 26.4669) -> (-363.7614, 30.0737) projected
  arc A222 (-363.2534, 30.5817) -> (-363.7614, 30.0737) centre (-363.2534, 30.0737) ccw projected
  line L255 (-363.2534, 30.5817) -> (-359.6466, 30.5817) projected
  arc A223 (-359.1386, 30.0737) -> (-359.6466, 30.5817) centre (-359.6466, 30.0737) ccw projected
  line L256 (-359.1386, 30.0737) -> (-359.1386, 26.4669) projected
  arc A224 (-359.6466, 25.9589) -> (-359.1386, 26.4669) centre (-359.6466, 26.4669) ccw projected
  line L257 (-359.6466, 25.9589) -> (-363.2534, 25.9589) projected
  arc A225 (-363.7614, 26.4669) -> (-363.2534, 25.9589) centre (-363.2534, 26.4669) ccw projected
  line L258 (-351.0614, 26.4669) -> (-351.0614, 30.0737) projected
  arc A226 (-350.5534, 30.5817) -> (-351.0614, 30.0737) centre (-350.5534, 30.0737) ccw projected
  line L259 (-350.5534, 30.5817) -> (-346.9466, 30.5817) projected
  arc A227 (-346.4386, 30.0737) -> (-346.9466, 30.5817) centre (-346.9466, 30.0737) ccw projected
  line L260 (-346.4386, 30.0737) -> (-346.4386, 26.4669) projected
  arc A228 (-346.9466, 25.9589) -> (-346.4386, 26.4669) centre (-346.9466, 26.4669) ccw projected
  line L261 (-346.9466, 25.9589) -> (-350.5534, 25.9589) projected
  arc A229 (-351.0614, 26.4669) -> (-350.5534, 25.9589) centre (-350.5534, 26.4669) ccw projected
  line L262 (-338.3614, 26.4669) -> (-338.3614, 30.0737) projected
  arc A230 (-337.8534, 30.5817) -> (-338.3614, 30.0737) centre (-337.8534, 30.0737) ccw projected
  line L263 (-337.8534, 30.5817) -> (-334.2466, 30.5817) projected
  arc A231 (-333.7386, 30.0737) -> (-334.2466, 30.5817) centre (-334.2466, 30.0737) ccw projected
  line L264 (-333.7386, 30.0737) -> (-333.7386, 26.4669) projected
  arc A232 (-334.2466, 25.9589) -> (-333.7386, 26.4669) centre (-334.2466, 26.4669) ccw projected
  line L265 (-334.2466, 25.9589) -> (-337.8534, 25.9589) projected
  arc A233 (-338.3614, 26.4669) -> (-337.8534, 25.9589) centre (-337.8534, 26.4669) ccw projected
  line L266 (-325.6614, 26.4669) -> (-325.6614, 30.0737) projected
  arc A234 (-325.1534, 30.5817) -> (-325.6614, 30.0737) centre (-325.1534, 30.0737) ccw projected
  line L267 (-325.1534, 30.5817) -> (-321.5466, 30.5817) projected
  arc A235 (-321.0386, 30.0737) -> (-321.5466, 30.5817) centre (-321.5466, 30.0737) ccw projected
  line L268 (-321.0386, 30.0737) -> (-321.0386, 26.4669) projected
  arc A236 (-321.5466, 25.9589) -> (-321.0386, 26.4669) centre (-321.5466, 26.4669) ccw projected
  line L269 (-321.5466, 25.9589) -> (-325.1534, 25.9589) projected
  arc A237 (-325.6614, 26.4669) -> (-325.1534, 25.9589) centre (-325.1534, 26.4669) ccw projected
  line L270 (-312.9614, 26.4669) -> (-312.9614, 30.0737) projected
  arc A238 (-312.4534, 30.5817) -> (-312.9614, 30.0737) centre (-312.4534, 30.0737) ccw projected
  line L271 (-312.4534, 30.5817) -> (-308.8466, 30.5817) projected
  arc A239 (-308.3386, 30.0737) -> (-308.8466, 30.5817) centre (-308.8466, 30.0737) ccw projected
  line L272 (-308.3386, 30.0737) -> (-308.3386, 26.4669) projected
  arc A240 (-308.8466, 25.9589) -> (-308.3386, 26.4669) centre (-308.8466, 26.4669) ccw projected
  line L273 (-308.8466, 25.9589) -> (-312.4534, 25.9589) projected
  arc A241 (-312.9614, 26.4669) -> (-312.4534, 25.9589) centre (-312.4534, 26.4669) ccw projected
  line L274 (-300.2614, 26.4669) -> (-300.2614, 30.0737) projected
  arc A242 (-299.7534, 30.5817) -> (-300.2614, 30.0737) centre (-299.7534, 30.0737) ccw projected
  line L275 (-299.7534, 30.5817) -> (-296.1466, 30.5817) projected
  arc A243 (-295.6386, 30.0737) -> (-296.1466, 30.5817) centre (-296.1466, 30.0737) ccw projected
  line L276 (-295.6386, 30.0737) -> (-295.6386, 26.4669) projected
  arc A244 (-296.1466, 25.9589) -> (-295.6386, 26.4669) centre (-296.1466, 26.4669) ccw projected
  line L277 (-296.1466, 25.9589) -> (-299.7534, 25.9589) projected
  arc A245 (-300.2614, 26.4669) -> (-299.7534, 25.9589) centre (-299.7534, 26.4669) ccw projected
  line L278 (-287.5614, 26.4669) -> (-287.5614, 30.0737) projected
  arc A246 (-287.0534, 30.5817) -> (-287.5614, 30.0737) centre (-287.0534, 30.0737) ccw projected
  line L279 (-287.0534, 30.5817) -> (-283.4466, 30.5817) projected
  arc A247 (-282.9386, 30.0737) -> (-283.4466, 30.5817) centre (-283.4466, 30.0737) ccw projected
  line L280 (-282.9386, 30.0737) -> (-282.9386, 26.4669) projected
  arc A248 (-283.4466, 25.9589) -> (-282.9386, 26.4669) centre (-283.4466, 26.4669) ccw projected
  line L281 (-283.4466, 25.9589) -> (-287.0534, 25.9589) projected
  arc A249 (-287.5614, 26.4669) -> (-287.0534, 25.9589) centre (-287.0534, 26.4669) ccw projected
  line L282 (-274.8614, 26.4669) -> (-274.8614, 30.0737) projected
  arc A250 (-274.3534, 30.5817) -> (-274.8614, 30.0737) centre (-274.3534, 30.0737) ccw projected
  line L283 (-274.3534, 30.5817) -> (-270.7466, 30.5817) projected
  arc A251 (-270.2386, 30.0737) -> (-270.7466, 30.5817) centre (-270.7466, 30.0737) ccw projected
  line L284 (-270.2386, 30.0737) -> (-270.2386, 26.4669) projected
  arc A252 (-270.7466, 25.9589) -> (-270.2386, 26.4669) centre (-270.7466, 26.4669) ccw projected
  line L285 (-270.7466, 25.9589) -> (-274.3534, 25.9589) projected
  arc A253 (-274.8614, 26.4669) -> (-274.3534, 25.9589) centre (-274.3534, 26.4669) ccw projected
  line L286 (-262.1614, 26.4669) -> (-262.1614, 30.0737) projected
  arc A254 (-261.6534, 30.5817) -> (-262.1614, 30.0737) centre (-261.6534, 30.0737) ccw projected
  line L287 (-261.6534, 30.5817) -> (-258.0466, 30.5817) projected
  arc A255 (-257.5386, 30.0737) -> (-258.0466, 30.5817) centre (-258.0466, 30.0737) ccw projected
  line L288 (-257.5386, 30.0737) -> (-257.5386, 26.4669) projected
  arc A256 (-258.0466, 25.9589) -> (-257.5386, 26.4669) centre (-258.0466, 26.4669) ccw projected
  line L289 (-258.0466, 25.9589) -> (-261.6534, 25.9589) projected
  arc A257 (-262.1614, 26.4669) -> (-261.6534, 25.9589) centre (-261.6534, 26.4669) ccw projected
  line L290 (-249.4614, 26.4669) -> (-249.4614, 30.0737) projected
  arc A258 (-248.9534, 30.5817) -> (-249.4614, 30.0737) centre (-248.9534, 30.0737) ccw projected
  line L291 (-248.9534, 30.5817) -> (-245.3466, 30.5817) projected
  arc A259 (-244.8386, 30.0737) -> (-245.3466, 30.5817) centre (-245.3466, 30.0737) ccw projected
  line L292 (-244.8386, 30.0737) -> (-244.8386, 26.4669) projected
  arc A260 (-245.3466, 25.9589) -> (-244.8386, 26.4669) centre (-245.3466, 26.4669) ccw projected
  line L293 (-245.3466, 25.9589) -> (-248.9534, 25.9589) projected
  arc A261 (-249.4614, 26.4669) -> (-248.9534, 25.9589) centre (-248.9534, 26.4669) ccw projected
  line L294 (-236.7614, 26.4669) -> (-236.7614, 30.0737) projected
  arc A262 (-236.2534, 30.5817) -> (-236.7614, 30.0737) centre (-236.2534, 30.0737) ccw projected
  line L295 (-236.2534, 30.5817) -> (-232.6466, 30.5817) projected
  arc A263 (-232.1386, 30.0737) -> (-232.6466, 30.5817) centre (-232.6466, 30.0737) ccw projected
  line L296 (-232.1386, 30.0737) -> (-232.1386, 26.4669) projected
  arc A264 (-232.6466, 25.9589) -> (-232.1386, 26.4669) centre (-232.6466, 26.4669) ccw projected
  line L297 (-232.6466, 25.9589) -> (-236.2534, 25.9589) projected
  arc A265 (-236.7614, 26.4669) -> (-236.2534, 25.9589) centre (-236.2534, 26.4669) ccw projected
  line L298 (-224.0614, 26.4669) -> (-224.0614, 30.0737) projected
  arc A266 (-223.5534, 30.5817) -> (-224.0614, 30.0737) centre (-223.5534, 30.0737) ccw projected
  line L299 (-223.5534, 30.5817) -> (-219.9466, 30.5817) projected
  arc A267 (-219.4386, 30.0737) -> (-219.9466, 30.5817) centre (-219.9466, 30.0737) ccw projected
  line L300 (-219.4386, 30.0737) -> (-219.4386, 26.4669) projected
  arc A268 (-219.9466, 25.9589) -> (-219.4386, 26.4669) centre (-219.9466, 26.4669) ccw projected
  line L301 (-219.9466, 25.9589) -> (-223.5534, 25.9589) projected
  arc A269 (-224.0614, 26.4669) -> (-223.5534, 25.9589) centre (-223.5534, 26.4669) ccw projected
  line L302 (-211.3614, 26.4669) -> (-211.3614, 30.0737) projected
  arc A270 (-210.8534, 30.5817) -> (-211.3614, 30.0737) centre (-210.8534, 30.0737) ccw projected
  line L303 (-210.8534, 30.5817) -> (-207.2466, 30.5817) projected
  arc A271 (-206.7386, 30.0737) -> (-207.2466, 30.5817) centre (-207.2466, 30.0737) ccw projected
  line L304 (-206.7386, 30.0737) -> (-206.7386, 26.4669) projected
  arc A272 (-207.2466, 25.9589) -> (-206.7386, 26.4669) centre (-207.2466, 26.4669) ccw projected
  line L305 (-207.2466, 25.9589) -> (-210.8534, 25.9589) projected
  arc A273 (-211.3614, 26.4669) -> (-210.8534, 25.9589) centre (-210.8534, 26.4669) ccw projected
  line L306 (-198.6614, 26.4669) -> (-198.6614, 30.0737) projected
  arc A274 (-198.1534, 30.5817) -> (-198.6614, 30.0737) centre (-198.1534, 30.0737) ccw projected
  line L307 (-198.1534, 30.5817) -> (-194.5466, 30.5817) projected
  arc A275 (-194.0386, 30.0737) -> (-194.5466, 30.5817) centre (-194.5466, 30.0737) ccw projected
  line L308 (-194.0386, 30.0737) -> (-194.0386, 26.4669) projected
  arc A276 (-194.5466, 25.9589) -> (-194.0386, 26.4669) centre (-194.5466, 26.4669) ccw projected
  line L309 (-194.5466, 25.9589) -> (-198.1534, 25.9589) projected
  arc A277 (-198.6614, 26.4669) -> (-198.1534, 25.9589) centre (-198.1534, 26.4669) ccw projected
  line L310 (-185.9614, 26.4669) -> (-185.9614, 30.0737) projected
  arc A278 (-185.4534, 30.5817) -> (-185.9614, 30.0737) centre (-185.4534, 30.0737) ccw projected
  line L311 (-185.4534, 30.5817) -> (-181.8466, 30.5817) projected
  arc A279 (-181.3386, 30.0737) -> (-181.8466, 30.5817) centre (-181.8466, 30.0737) ccw projected
  line L312 (-181.3386, 30.0737) -> (-181.3386, 26.4669) projected
  arc A280 (-181.8466, 25.9589) -> (-181.3386, 26.4669) centre (-181.8466, 26.4669) ccw projected
  line L313 (-181.8466, 25.9589) -> (-185.4534, 25.9589) projected
  arc A281 (-185.9614, 26.4669) -> (-185.4534, 25.9589) centre (-185.4534, 26.4669) ccw projected
  line L314 (-173.2614, 26.4669) -> (-173.2614, 30.0737) projected
  arc A282 (-172.7534, 30.5817) -> (-173.2614, 30.0737) centre (-172.7534, 30.0737) ccw projected
  line L315 (-172.7534, 30.5817) -> (-169.1466, 30.5817) projected
  arc A283 (-168.6386, 30.0737) -> (-169.1466, 30.5817) centre (-169.1466, 30.0737) ccw projected
  line L316 (-168.6386, 30.0737) -> (-168.6386, 26.4669) projected
  arc A284 (-169.1466, 25.9589) -> (-168.6386, 26.4669) centre (-169.1466, 26.4669) ccw projected
  line L317 (-169.1466, 25.9589) -> (-172.7534, 25.9589) projected
  arc A285 (-173.2614, 26.4669) -> (-172.7534, 25.9589) centre (-172.7534, 26.4669) ccw projected
  line L318 (-160.5614, 26.4669) -> (-160.5614, 30.0737) projected
  arc A286 (-160.0534, 30.5817) -> (-160.5614, 30.0737) centre (-160.0534, 30.0737) ccw projected
  line L319 (-160.0534, 30.5817) -> (-156.4466, 30.5817) projected
  arc A287 (-155.9386, 30.0737) -> (-156.4466, 30.5817) centre (-156.4466, 30.0737) ccw projected
  line L320 (-155.9386, 30.0737) -> (-155.9386, 26.4669) projected
  arc A288 (-156.4466, 25.9589) -> (-155.9386, 26.4669) centre (-156.4466, 26.4669) ccw projected
  line L321 (-156.4466, 25.9589) -> (-160.0534, 25.9589) projected
  arc A289 (-160.5614, 26.4669) -> (-160.0534, 25.9589) centre (-160.0534, 26.4669) ccw projected
  line L322 (-147.8614, 26.4669) -> (-147.8614, 30.0737) projected
  arc A290 (-147.3534, 30.5817) -> (-147.8614, 30.0737) centre (-147.3534, 30.0737) ccw projected
  line L323 (-147.3534, 30.5817) -> (-143.7466, 30.5817) projected
  arc A291 (-143.2386, 30.0737) -> (-143.7466, 30.5817) centre (-143.7466, 30.0737) ccw projected
  line L324 (-143.2386, 30.0737) -> (-143.2386, 26.4669) projected
  arc A292 (-143.7466, 25.9589) -> (-143.2386, 26.4669) centre (-143.7466, 26.4669) ccw projected
  line L325 (-143.7466, 25.9589) -> (-147.3534, 25.9589) projected
  arc A293 (-147.8614, 26.4669) -> (-147.3534, 25.9589) centre (-147.3534, 26.4669) ccw projected
  line L326 (-135.1614, 26.4669) -> (-135.1614, 30.0737) projected
  arc A294 (-134.6534, 30.5817) -> (-135.1614, 30.0737) centre (-134.6534, 30.0737) ccw projected
  line L327 (-134.6534, 30.5817) -> (-131.0466, 30.5817) projected
  arc A295 (-130.5386, 30.0737) -> (-131.0466, 30.5817) centre (-131.0466, 30.0737) ccw projected
  line L328 (-130.5386, 30.0737) -> (-130.5386, 26.4669) projected
  arc A296 (-131.0466, 25.9589) -> (-130.5386, 26.4669) centre (-131.0466, 26.4669) ccw projected
  line L329 (-131.0466, 25.9589) -> (-134.6534, 25.9589) projected
  arc A297 (-135.1614, 26.4669) -> (-134.6534, 25.9589) centre (-134.6534, 26.4669) ccw projected
  line L330 (-416.7966, 20.1169) -> (-420.4034, 23.7237) construction
  line L331 (-418.6, 21.9203) -> (-418.6, -44.1197) construction
  line L332 (-418.6, 21.9203) -> (-352.56, 21.9203) construction
  line L333 (-418.6, -44.1197) -> (-363.8737, 10.6066)
  line L334 (-418.6, -44.1197) -> (-341.2053, -44.1197) construction
  line L335 (-363.8737, 21.9203) -> (-437.9137, -52.1197)
  line L336 (-437.9137, -52.1197) -> (-321.0323, -52.1197)
  line L337 (-418.6, -44.1197) -> (-424.2569, -38.4628)
  line L338 (-363.8737, 10.6066) -> (-363.8737, 21.9203)
  line L339 (-375.9534, 30.0737) -> (-372.3466, 26.4669) construction
  line L340 (-382.3034, 23.7237) -> (-378.6966, 20.1169) construction
  line L341 (-388.6534, 17.3737) -> (-385.0466, 13.7669) construction
  circle A298 centre (-386.85, 15.5703) radius 2.159
  circle A299 centre (-380.5, 21.9203) radius 2.159
  circle A300 centre (-374.15, 28.2703) radius 2.159
  line L342 (-386.85, 15.5703) -> (-374.15, 28.2703) construction
  line L343 (-383.2579, 11.9782) -> (-370.5579, 24.6782)
  line L344 (-377.7421, 31.8624) -> (-390.4421, 19.1624)
  arc A301 (-390.4421, 19.1624) -> (-383.2579, 11.9782) centre (-386.85, 15.5703) ccw
  arc A302 (-370.5579, 24.6782) -> (-377.7421, 31.8624) centre (-374.15, 28.2703) ccw
  line L345 (-363.8737, 21.9203) -> (-369.9099, 31.0681)
  line L346 (-421.4284, -41.2913) -> (-363.8737, 16.2634) construction
  line L347 (-418.6, -38.4628) -> (-400.6395, -20.5023) construction
  line L348 (-417.504, -39.5589) -> (-399.5435, -21.5984)
  line L349 (-401.7355, -19.4063) -> (-419.696, -37.3668)
  arc A303 (-419.696, -37.3668) -> (-417.504, -39.5589) centre (-418.6, -38.4628) ccw
  arc A304 (-399.5435, -21.5984) -> (-401.7355, -19.4063) centre (-400.6395, -20.5023) ccw
  line L350 (-400.6395, -20.5023) -> (-382.679, -2.5418) construction
  line L351 (-382.679, -2.5418) -> (-369.2086, 10.9286) construction
  line L352 (-381.583, -3.6378) -> (-368.1126, 9.8325)
  line L353 (-370.3046, 12.0246) -> (-383.775, -1.4458)
  arc A305 (-383.775, -1.4458) -> (-381.583, -3.6378) centre (-382.679, -2.5418) ccw
  arc A306 (-368.1126, 9.8325) -> (-370.3046, 12.0246) centre (-369.2086, 10.9286) ccw
  line L354 (-391.93, 15.5703) -> (-391.93, -6.136)
  circle A307 centre (-391.6592, -11.5221) radius 2.159
  point P0 (0, 0)
  point P1 (-380.5, 21.9203)
  point P2 (-409.6197, -29.4826)
  point P3 (-375.9438, 4.1934)
  point P4 (-370.971, 32.2327)
  point P5 (-377.329, 32.2327)
  dimension "d0" = 66.04
  dimension "d1" = 90
  dimension "d2" = 45
  dimension "d3" = 8
  dimension "d4" = 4.318
  dimension "d5" = 10.16
  dimension "d6" = 25.4
  dimension "d7" = 3.1
  dimension "d8" = 25.4
  dimension "d9" = 19.05
  dimension "d10" = 4.318
  constraints: 56 end point, 14 point on circle, 14 tangent, 10 centre point, 10 midpoint, 8 point on line, 3 equal radius, 3 parallel, 3 vertical, 2 equal length, 2 horizontal, 2 perpendicular, 1 coincident, 1 vertical alignment, 1 other
  measures "d0" distance of L331.start L331.end
  measures "d1" angle of L331 L332
  measures "d2" angle of L334 L333
  measures "d3" distance between parallel lines of L333 L335
  measures "d4" diameter of A298
  measures "d5" diameter of A302
  measures "d6" distance of L347.start L347.end
  measures "d7" diameter of A304
  measures "d8" distance of L347.end L350.end
  measures "d9" distance of L350.end L351.end
  measures "d10" diameter of A307
extrude "Extrusion1" add sketch "Sketch1" along normal blind 3 contours L16 A16 L17 A17 L18 A18 L19 A19 | A23 L23 A22 L22 A21 L21 L335 L156 A123 L155 A122 L154 A125 L157 L119 L118 L117 L116 A301 L343 A302 L345 L20 | L20 L335 L21 A21 L22 A22 L23 A23 | L335 L338 L119 A306 L353 L157 A124 L156 L21 A20 L20 | L20 A20 L21 L335 | L338 L333 L337 L335 L119 L353 A305 L352 A306 | A302 L343 A301 L116 L344 L111 | L335 L157 A125 L154 A122 L155 A123 L156 | L156 A124 L157 L335 | L335 L354 L116 A301 L117 L118 L119 | A301 L116 | L116 L354 A301 | L150 A118 L151 A119 L152 A120 L153 A121 | L250 A218 L251 A219 L252 A220 L253 A221
fillet "Fillet1" radius 2.5 6 edges at (-370.971, 32.2327, 1.5) (-377.329, 32.2327, 1.5) (-363.8737, 21.9203, 1.5) (-363.8737, 10.6066, 1.5) (-424.2569, -38.4628, 1.5) (-418.6, -44.1197, 1.5)
fillet "Fillet2" radius 25.4 1 edges at (-391.93, -6.136, 1.5)